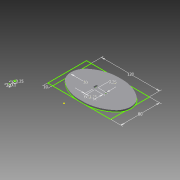
# Autodesk Inventor part: body-back
Saved by Autodesk Inventor 2013 (Build 170138000, 138)
## iProperties
Created: 2012-09-08
Part Number: body-back
Material: Generic
Document SubType Name: Modeling
Designer: frankenteddy
Density: 1 g/cm^3
Author: frankenteddy
Autodesk Inventor part; units mm, degrees
ref_plane "YZ Plane" through (0, 0, 0) normal (1, 0, 0) x (0, 1, 0)
ref_plane "XZ Plane" through (0, 0, 0) normal (0, 1, 0) x (-1, 0, 0)
ref_plane "XY Plane" through (0, 0, 0) normal (0, 0, 1) x (1, 0, 0)
sketch "Sketch1" plane through (0, 0, 0) normal (0, 0, 1) x (1, 0, 0)
  line L0 (-92.7646, -8.503) -> (-89.7646, -8.503)
  line L1 (-89.7646, -8.503) -> (-89.7646, -11.753)
  line L2 (-89.7646, -11.753) -> (-92.7646, -11.753)
  line L3 (-92.7646, -11.753) -> (-92.7646, -8.503)
  line L4 (-92.7646, -21.6527) -> (-89.7646, -21.6527)
  line L5 (-89.7646, -21.6527) -> (-89.7646, -21.7527)
  line L6 (-89.7646, -21.7527) -> (-92.7646, -21.7527)
  line L7 (-92.7646, -21.7527) -> (-92.7646, -21.6527)
  line L8 (-43.5121, 19.6165) -> (76.4879, 19.6165)
  line L9 (76.4879, 19.6165) -> (76.4879, 99.6165)
  line L10 (76.4879, 99.6165) -> (-43.5121, 99.6165)
  line L11 (-43.5121, 99.6165) -> (-43.5121, 19.6165)
  line L12 (16.4879, 99.6165) -> (16.4879, 19.6165) construction
  line L13 (-43.5121, 59.6165) -> (76.4879, 59.6165) construction
  line L14 (3.9879, 63.1165) -> (7.2379, 63.1165)
  line L15 (7.2379, 63.1165) -> (7.2379, 56.1165)
  line L16 (7.2379, 56.1165) -> (3.9879, 56.1165)
  line L17 (3.9879, 56.1165) -> (3.9879, 63.1165)
  line L18 (3.9879, 59.6165) -> (7.2379, 59.6165) construction
  line L19 (28.9879, 63.1165) -> (25.7379, 63.1165)
  line L20 (25.7379, 63.1165) -> (25.7379, 56.1165)
  line L21 (25.7379, 56.1165) -> (28.9879, 56.1165)
  line L22 (28.9879, 56.1165) -> (28.9879, 63.1165)
  line L23 (28.9879, 59.6165) -> (25.7379, 59.6165) construction
  line L24 (-43.5121, 99.6165) -> (-53.5121, 99.6165)
  line L25 (-53.5121, 99.6165) -> (-53.5121, 19.6165)
  line L26 (-53.5121, 19.6165) -> (-43.5121, 19.6165)
  line L27 (-43.5121, 19.6165) -> (-43.5121, 99.6165)
  arc A0 (16.4879, 99.6165) -> (-34.1013, 83.0147) centre (13.3048, 23.9368) ccw
  arc A1 (-34.1013, 36.2182) -> (16.4879, 19.6165) centre (13.3048, 95.2961) ccw
  arc A2 (-34.1013, 83.0147) -> (-34.1013, 36.2182) centre (-15.3258, 59.6165) ccw
  arc A3 (67.0771, 83.0147) -> (16.4879, 99.6165) centre (19.6709, 23.9368) ccw
  arc A4 (16.4879, 19.6165) -> (67.0771, 36.2182) centre (19.6709, 95.2961) ccw
  arc A5 (67.0771, 36.2182) -> (67.0771, 83.0147) centre (48.3015, 59.6165) ccw
  point P0 (0, 0)
  point P1 (-10.3135, 95.9071)
  point P2 (-37.4785, 79.8466)
  dimension "d3" = 3
  dimension "mat" = 3.25
  dimension "d5" = 3
  dimension "kerf" = 0.1
  dimension "d42" = 120
  dimension "d43" = 80
  dimension "d44" = 3.25
  dimension "d45" = 7
  dimension "d47" = 9.25
  dimension "d69" = 10
  dimension "d70" = 30
  constraints: 56 end point, 14 point on circle, 12 symmetric about line, 10 parallel, 6 centre point, 6 midpoint, 5 horizontal, 5 perpendicular, 2 tangent, 1 collinear, 4 other
  measures "d3" distance of L1.end L2.end
  measures "mat" distance of L0.end L1.end
  measures "d5" distance of L5.end L6.end
  measures "kerf" distance of L4.end L5.end
  measures "d42" distance of L10.end L9.end
  measures "d43" distance of L9.end L8.end
  measures "d44" distance of L15.end L16.end
  measures "d45" distance of L14.end L15.end
  measures "d47" distance between parallel lines of L12 L15
  measures "d69" distance of L26.end L25.end
  measures "d70" radius of A2
extrude "Extrusion10" add sketch "Sketch1" along normal blind 3.25 contours A1 A2 L11 A0 L10 A3 A5 L9 A4 L8 | L8 A1 | A2 L11 | L8 A4 | A0 L10 | L9 A5 | A3 L10
equation "\"d44\" = mat"
equation "\"d73\" = mat"
body "Solid4"
